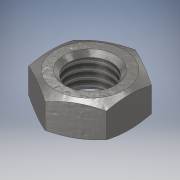
# Autodesk Inventor part: porca m3
Saved by Autodesk Inventor 2019.4 (Build 234330000, 330)
## iProperties
Created: 2021-02-09
Part Number: porca m3
Material: Aço galvanizado
Document SubType Name: Modeling
Designer: Lattes
Density: 7.85 g/cm^3
Appearance: Galvanizado
Author: Lattes
Autodesk Inventor part; units mm, degrees
ref_plane "YZ Plane" through (0, 0, 0) normal (1, 0, 0) x (0, 1, 0)
ref_plane "XZ Plane" through (0, 0, 0) normal (0, 1, 0) x (-1, 0, 0)
ref_plane "XY Plane" through (0, 0, 0) normal (0, 0, 1) x (1, 0, 0)
sketch "Esboço2" plane through (0, 0, 0) normal (0, 1, 0) x (-1, 0, 0)
  circle A0 centre (0, 0) radius 1.5
  line L0 (2.7, -1.5588) -> (0, -3.1177)
  line L1 (0, -3.1177) -> (-2.7, -1.5588)
  line L2 (-2.7, -1.5588) -> (-2.7, 1.5588)
  line L3 (-2.7, 1.5588) -> (0, 3.1177)
  line L4 (0, 3.1177) -> (2.7, 1.5588)
  line L5 (2.7, 1.5588) -> (2.7, -1.5588)
  constraints: 12 end point, 1 centre point
extrude "Extrusão1" add sketch "Esboço2" along normal blind 2.4
thread "Rosca1" size "M3x0.5" class "6H" standard "ANSI Metric M Profile" full length
chamfer "Chanfro1" distance 0.3 angle 45 2 edges at (1.5, 2.4, 0) (1.5, 0, 0)
sketch "Esboço3" plane through (0, 0, 0) normal (0, 0, 1) x (1, 0, 0)
  line L0 (0, -0.6576) -> (0, 3.9457) projected
  line L1 (2.4, 2.4) -> (4.5158, 1.4134)
  line L2 (2.4, 2.4) -> (4.7345, 2.4) construction
  line L3 (2.4, 0) -> (4.5158, 0.9866)
  line L4 (2.4, 2.4) -> (4.5158, 2.4)
  line L5 (2.4, 0) -> (4.5158, 0.9866)
  line L6 (2.4, 2.4) -> (4.5158, 1.4134)
  line L7 (4.5158, 1.4134) -> (4.5158, 2.4)
  line L8 (4.5158, 0.9866) -> (4.5158, 0)
  line L9 (4.5158, 0.9866) -> (2.4, 0)
  line L10 (2.4, 0) -> (4.5158, 0)
  line L11 (2.7, 0) -> (0, 0) projected
  dimension "d16" = 25
  constraints: 20 end point, 3 collinear, 1 equal length, 1 horizontal, 1 point on line, 1 vertical
  measures "d16" angle of L1 L2
revolve "Revolução2" cut sketch "Esboço3" angle 360 about axis through (0, -10, 0) along (0, 1, 0)
